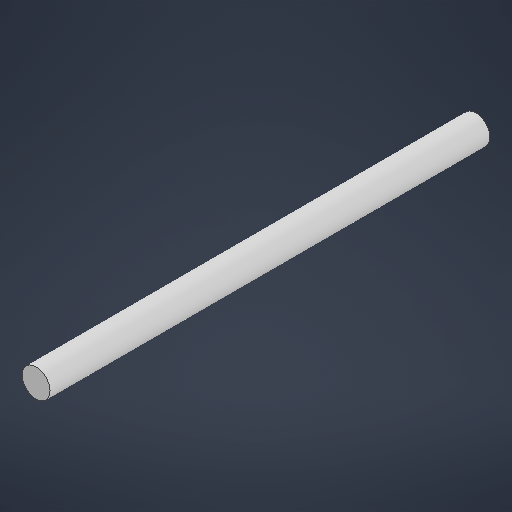
# Autodesk Inventor part: Porsche_912_Main_CV_Shaft
Saved by Autodesk Inventor 2026.1 (Build 301233000, 233)
## iProperties
Created: 2026-08-06
Part Number: Porsche_912_Main_CV_Shaft
Material: Generic
Document SubType Name: Modeling
Designer: share
Density: 1 g/cm^3
Appearance: Default
Mass: 202.683 g
Surface Area: 329.32 cm^2
Volume: 202.683 cm^3
Author: share
Autodesk Inventor part; units mm, degrees
ref_plane "YZ Plane" through (0, 0, 0) normal (1, 0, 0) x (0, 1, 0)
ref_plane "XZ Plane" through (0, 0, 0) normal (0, 1, 0) x (-1, 0, 0)
ref_plane "XY Plane" through (0, 0, 0) normal (0, 0, 1) x (1, 0, 0)
sketch "Sketch1" plane through (0, 0, 0) normal (1, 0, 0) x (0, 1, 0)
  line L0 (0, 200) -> (0, -200)
  line L1 (0, -185) -> (0, 185) construction
  line L2 (0, 200) -> (12.7, 200)
  line L3 (12.7, 200) -> (12.7, -200)
  line L4 (12.7, -200) -> (0, -200)
  point P0 (0, 0)
  dimension "d0" = 400
  dimension "d1" = 370
  dimension "d4" = 12.7
  constraints: 10 end point, 2 coincident, 2 midpoint, 2 perpendicular, 2 vertical, 1 horizontal
  measures "d0" distance of L0.start L0.end
  measures "d1" distance of L1.start L1.end
  measures "d4" distance between parallel lines of L1 L3
revolve "Revolution1" add sketch "Sketch1" angle 360 about axis through (0, 0, 200) along (0, 0, -1)
body "Solid1"
